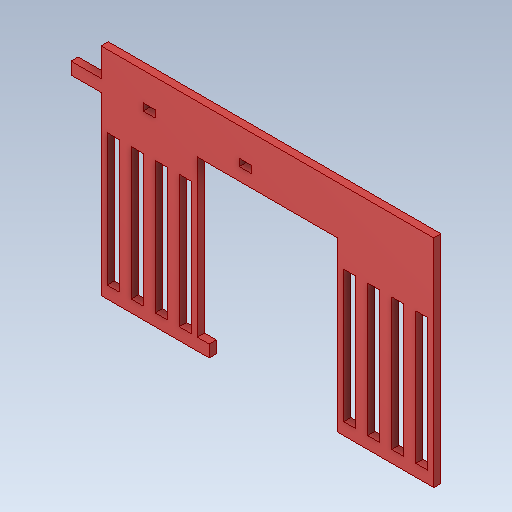
# Autodesk Inventor part: Celda puertas
Saved by Autodesk Inventor 2020 (Build 240168000, 168)
## iProperties
Created: 2020-03-12
Part Number: Celda puertas
Material: Genérico
Document SubType Name: Modeling
Designer: joser
Density: 1 g/cm^3
Appearance: Suave - Rojo
Author: joser
Autodesk Inventor part; units mm, degrees
ref_plane "YZ Plane" through (0, 0, 0) normal (1, 0, 0) x (0, 1, 0)
ref_plane "XZ Plane" through (0, 0, 0) normal (0, 1, 0) x (-1, 0, 0)
ref_plane "XY Plane" through (0, 0, 0) normal (0, 0, 1) x (1, 0, 0)
sketch "Boceto1" plane through (0, 0, 0) normal (0, 0, 1) x (1, 0, 0)
  line L0 (40, 70) -> (40, 5)
  line L1 (2.5, 60) -> (7.5, 60)
  line L2 (7.5, 60) -> (7.5, 5)
  line L3 (7.5, 5) -> (2.5, 5)
  line L4 (2.5, 5) -> (2.5, 60)
  line L5 (12.5, 60) -> (17.5, 60)
  line L6 (17.5, 60) -> (17.5, 5)
  line L7 (17.5, 5) -> (12.5, 5)
  line L8 (12.5, 5) -> (12.5, 60)
  line L9 (22.5, 60) -> (27.5, 60)
  line L10 (27.5, 60) -> (27.5, 5)
  line L11 (27.5, 5) -> (22.5, 5)
  line L12 (22.5, 5) -> (22.5, 60)
  line L13 (32.5, 60) -> (37.5, 60)
  line L14 (37.5, 60) -> (37.5, 5)
  line L15 (37.5, 5) -> (32.5, 5)
  line L16 (32.5, 5) -> (32.5, 60)
  line L17 (138.5, 90) -> (138.5, 0)
  line L18 (138.5, 0) -> (98.5, 0)
  line L19 (98.5, 0) -> (98.5, 70)
  line L20 (101, 60) -> (106, 60)
  line L21 (106, 60) -> (106, 5)
  line L22 (106, 5) -> (101, 5)
  line L23 (101, 5) -> (101, 60)
  line L24 (111, 60) -> (116, 60)
  line L25 (116, 60) -> (116, 5)
  line L26 (116, 5) -> (111, 5)
  line L27 (111, 5) -> (111, 60)
  line L28 (121, 60) -> (126, 60)
  line L29 (126, 60) -> (126, 5)
  line L30 (126, 5) -> (121, 5)
  line L31 (121, 5) -> (121, 60)
  line L32 (136, 60) -> (136, 5)
  line L33 (131, 5) -> (131, 60)
  line L34 (131, 60) -> (136, 60)
  line L35 (136, 5) -> (131, 5)
  line L36 (0, 90) -> (138.5, 90)
  line L37 (40, 70) -> (98.5, 70)
  line L38 (17.5, 78.25) -> (22.5, 78.25)
  line L39 (22.5, 78.25) -> (22.5, 75.25)
  line L40 (22.5, 75.25) -> (17.5, 75.25)
  line L41 (17.5, 75.25) -> (17.5, 78.25)
  line L42 (20, 78.25) -> (20, 75.25) construction
  line L43 (17.5, 76.75) -> (22.5, 76.75) construction
  line L44 (57.5, 78.25) -> (62.5, 78.25)
  line L45 (62.5, 78.25) -> (62.5, 75.25)
  line L46 (62.5, 75.25) -> (57.5, 75.25)
  line L47 (57.5, 75.25) -> (57.5, 78.25)
  line L48 (60, 78.25) -> (60, 75.25) construction
  line L49 (57.5, 76.75) -> (62.5, 76.75) construction
  line L50 (45, 0) -> (45, 5)
  line L51 (45, 5) -> (40, 5)
  line L52 (45, 0) -> (0, 0)
  line L53 (0, 78.25) -> (-12.5, 78.25)
  line L54 (-12.5, 78.25) -> (-12.5, 73.25)
  line L55 (-12.5, 73.25) -> (0, 73.25)
  line L56 (0, 0) -> (0, 73.25)
  line L57 (0, 78.25) -> (0, 90)
  point P0 (0, 0)
  dimension "d46" = 5
  dimension "d85" = 5
  dimension "d86" = 5
  dimension "d87" = 5
  dimension "d89" = 40
  dimension "d90" = 5
  dimension "d94" = 5
  dimension "d95" = 5
  dimension "d96" = 5
  dimension "d112" = 2.5
  dimension "d120" = 5
  dimension "d121" = 3
  dimension "d134" = 5
  dimension "d135" = 3
  dimension "d136" = 35
  dimension "d141" = 5
  dimension "d145" = 55
  dimension "d155" = 70
  dimension "d156" = 90
  dimension "d157" = 76.75
  dimension "d158" = 5
  dimension "d161" = 5
  dimension "d162" = 40
  dimension "d163" = 2.5
  dimension "d164" = 138.5
  dimension "d165" = 20
  dimension "d166" = 12.5
  constraints: 116 end point, 23 parallel, 15 perpendicular, 13 equal length, 12 collinear, 12 horizontal, 8 midpoint, 1 coincident
  measures "d46" distance of L2.end L3.end
  measures "d85" distance between parallel lines of L8 L2
  measures "d86" distance between parallel lines of L12 L6
  measures "d87" distance between parallel lines of L16 L10
  measures "d89" distance of L17.end L19.start
  measures "d90" distance of L21.end L23.start
  measures "d94" distance between parallel lines of L27 L21
  measures "d95" distance between parallel lines of L31 L25
  measures "d96" distance between parallel lines of L33 L29
  measures "d112" distance between parallel lines of L19 L23
  measures "d120" distance of L39.end L40.end
  measures "d121" distance of L38.end L39.end
  measures "d134" distance of L46.start L46.end
  measures "d135" distance of L45.start L46.start
  measures "d136" distance between parallel lines of L47 L39
  measures "d141" distance between parallel lines of L0 L50
  measures "d145" distance between parallel lines of L51 L13
  measures "d155" distance between parallel lines of L18 L37
  measures "d156" distance between parallel lines of L52 L36
  measures "d157" distance between parallel lines of L52 L43
  measures "d158" distance between parallel lines of L52 L51
  measures "d161" distance between parallel lines of L55 L53
  measures "d162" distance between parallel lines of L56 L0
  measures "d163" distance between parallel lines of L56 L4
  measures "d164" distance between parallel lines of L17 L56
  measures "d165" distance between parallel lines of L57 L42
  measures "d166" distance between parallel lines of L57 L54
extrude "Extrusión7" add sketch "Boceto1" along normal blind 3
